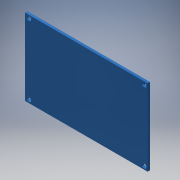
# Autodesk Inventor part: screen
Saved by Autodesk Inventor 2017 (Build 210142000, 142)
## iProperties
Part Number: screen
Material: Genérico
Document SubType Name: Modeling
Designer: Roberto
Density: 1 g/cm^3
Appearance: Valor por defecto
Author: Roberto
Autodesk Inventor part; units mm, degrees
ref_plane "YZ Plane" through (0, 0, 0) normal (1, 0, 0) x (0, 1, 0)
ref_plane "XZ Plane" through (0, 0, 0) normal (0, 1, 0) x (-1, 0, 0)
sketch "Boceto6" plane through (0, 0, 0) normal (0, 1, 0) x (-1, 0, 0)
  line L0 (0, 0) -> (9.64, 0)
  line L1 (9.64, 0) -> (9.64, -6.006)
  line L2 (9.64, -6.006) -> (0, -6.006)
  line L3 (0, -6.006) -> (0, 0)
  arc A0 (0.25, -0.1) -> (0.25, -0.4) centre (0.25, -0.25) ccw
  arc A1 (0.35, -0.4) -> (0.35, -0.1) centre (0.35, -0.25) ccw
  line L4 (0.25, -0.4) -> (0.35, -0.4)
  line L5 (0.25, -0.1) -> (0.35, -0.1)
  arc A2 (9.29, -0.1) -> (9.29, -0.4) centre (9.29, -0.25) ccw
  arc A3 (9.39, -0.4) -> (9.39, -0.1) centre (9.39, -0.25) ccw
  line L6 (9.29, -0.4) -> (9.39, -0.4)
  line L7 (9.29, -0.1) -> (9.39, -0.1)
  arc A4 (0.25, -5.906) -> (0.25, -5.906) centre (0.25, -5.946) ccw
  arc A5 (0.35, -5.906) -> (0.35, -5.906) centre (0.2, -5.906) ccw
  line L8 (0.25, -5.906) -> (0.35, -5.906)
  line L9 (0.25, -5.906) -> (0.35, -5.906)
  arc A6 (9.29, -5.906) -> (9.29, -5.906) centre (9.29, -5.756) ccw
  arc A7 (9.39, -5.906) -> (9.39, -5.906) centre (9.39, -5.946) ccw
  line L10 (9.29, -5.906) -> (9.39, -5.906)
  line L11 (9.29, -5.906) -> (9.39, -5.906)
  arc A8 (0.25, -5.606) -> (0.25, -5.906) centre (0.25, -5.756) ccw
  arc A9 (0.35, -5.906) -> (0.35, -5.606) centre (0.35, -5.756) ccw
  line L12 (0.25, -5.906) -> (0.35, -5.906)
  line L13 (0.25, -5.606) -> (0.35, -5.606)
  arc A10 (9.29, -5.606) -> (9.29, -5.906) centre (9.29, -5.756) ccw
  arc A11 (9.39, -5.906) -> (9.39, -5.606) centre (9.39, -5.756) ccw
  line L14 (9.29, -5.906) -> (9.39, -5.906)
  line L15 (9.29, -5.606) -> (9.39, -5.606)
  dimension "d33" = 9.64
  dimension "d34" = 0.25
  dimension "d35" = 0.1
  dimension "d36" = 0.25
  dimension "d37" = 0.25
  dimension "d41" = 6.006
  dimension "d42" = 0.1
  dimension "d43" = 0.1
  dimension "d44" = 0.1
  dimension "d45" = 0.1
  constraints: 32 end point, 24 point on circle, 12 centre point
  measures "d33" distance between parallel lines of L3 L1
  measures "d34" distance from line of L3 A4.centre
  measures "d35" distance edge to line of A0 L3
  measures "d36" distance from line of L1 A3.centre
  measures "d37" distance from line of L1 A7.centre
  measures "d41" distance between parallel lines of L0 L2
  measures "d42" distance between parallel lines of L2 L10
  measures "d43" distance between parallel lines of L2 L8
  measures "d44" distance between parallel lines of L0 L5
  measures "d45" distance between parallel lines of L0 L7
extrude "Extrusión4" add sketch "Boceto6" along normal blind 0.2 contours L0 L1 L2 A5 A9 L13 A8 L3 | A4 | A5 A8 L8 L2 | A7
sketch "Boceto7" plane through (0, 0.2, 0) normal (0, 1, 0) x (1, 0, 0)
  line L0 (-9.29, 0.1) -> (-9.39, 0.1) projected
  arc A0 (-9.39, 0.4) -> (-9.39, 0.1) centre (-9.39, 0.25) ccw projected
  line L1 (-9.39, 0.4) -> (-9.29, 0.4) projected
  arc A1 (-9.29, 0.1) -> (-9.29, 0.4) centre (-9.29, 0.25) ccw projected
  line L2 (-0.25, 0.1) -> (-0.35, 0.1) projected
  arc A2 (-0.35, 0.4) -> (-0.35, 0.1) centre (-0.35, 0.25) ccw projected
  line L3 (-0.35, 0.4) -> (-0.25, 0.4) projected
  arc A3 (-0.25, 0.1) -> (-0.25, 0.4) centre (-0.25, 0.25) ccw projected
  line L4 (-9.64, 0) -> (0, 0) projected
  line L5 (0, 0) -> (0, 6.006) projected
  line L6 (0, 6.006) -> (-9.64, 6.006) projected
  line L7 (-9.64, 6.006) -> (-9.64, 0) projected
  line L8 (-9.64, 6.006) -> (0, 6.006) projected
  line L9 (0, 0) -> (0, 6.006) projected
  line L10 (-0.8, 5.546) -> (-0.8, 0.65)
  line L11 (-0.8, 0.65) -> (-8.74, 0.65)
  line L12 (-8.74, 0.65) -> (-8.74, 5.546)
  line L13 (-8.74, 5.546) -> (-0.8, 5.546)
  dimension "d39" = 7.94
  dimension "d40" = 0.8
  constraints: 8 end point
  measures "d39" distance of L13.start L10.start
  measures "d40" distance between parallel lines of L5 L10
extrude "Extrusión5" cut sketch "Boceto7" along normal blind 0.4 contours L10 L11 L12 L13
ref_plane "Plano de trabajo2" through (0, 2.3, 0) normal (0, 1, 0) x (1, 0, 0)
sketch "Boceto9" plane through (0, 2.3, 0) normal (0, 1, 0) x (1, 0, 0)
  line L0 (-8.9922, 5.6013) -> (-0.8, 5.6013) construction
  line L1 (-0.8, 5.6013) -> (-0.8, 0.65) construction
  line L2 (-0.8, 0.65) -> (-8.9922, 0.65) construction
  line L3 (-8.9922, 0.65) -> (-8.9922, 5.6013) construction
  line L4 (-0.8, 5.546) -> (-8.74, 5.546) projected
  line L5 (-8.74, 5.546) -> (-8.74, 0.65) projected
  line L6 (-8.74, 0.65) -> (-0.8, 0.65) projected
  line L7 (-0.8, 0.65) -> (-0.8, 5.546) projected
  point P0 (0, 0)
  constraints: 2 other
decal "Calcomanía1"
